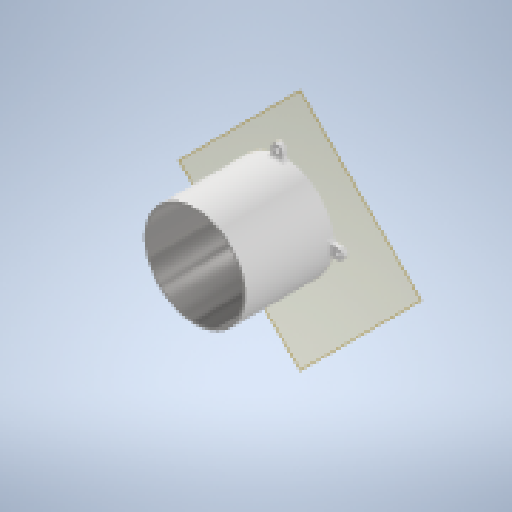
# Autodesk Inventor part: Camisa
Saved by Autodesk Inventor 2023 (Build 270158000, 158)
## iProperties
Created: 2022-11-24
Part Number: Camisa
Material: Genérico
Document SubType Name: Modeling
Designer: sergi
Density: 1 g/cm^3
Appearance: Valor por defecto
Author: sergi
Autodesk Inventor part; units mm, degrees
ref_plane "YZ Plane" through (0, 0, 0) normal (1, 0, 0) x (0, 1, 0)
ref_plane "XZ Plane" through (0, 0, 0) normal (0, 1, 0) x (-1, 0, 0)
ref_plane "XY Plane" through (0, 0, 0) normal (0, 0, 1) x (1, 0, 0)
ref_plane "Plano de trabajo1" through (0, 0, 0) normal (0, 0, 1) x (1, 0, 0)
sketch "Boceto1" plane through (0, 0, 0) normal (0, 0, 1) x (1, 0, 0)
  arc A0 (29.505692, -74.908522) -> (70.494308, -74.908522) centre (50, -53) ccw
  circle A1 centre (50, -53) radius 30
  circle A2 centre (50, -53) radius 31.5
  point P0 (0, 0)
  dimension "d0" = 60
  dimension "d1" = 63
  constraints: 2 centre point, 2 coincident
  measures "d0" diameter of A1
  measures "d1" diameter of A2
extrude "Extrusión1" add sketch "Boceto1" along normal blind 55
ref_plane "Plano de trabajo2" through (38.332738, -41.332738, 0) normal (0, 0, 1) x (0.7071068, 0.7071068, 0)
sketch "Boceto3" plane through (38.332738, -41.332738, 0) normal (0, 0, 1) x (0.7071068, 0.7071068, 0)
  circle A0 centre (25.37, -43.5) radius 1.25
  arc A1 (23.001522, -45.725492) -> (27.738478, -41.274508) centre (25.37, -43.5) ccw
  line L0 (-2.057062, -23.435368) -> (-6.794017, -18.984385)
  circle A2 centre (-25.37, -43.5) radius 1.25
  arc A3 (-27.738478, -41.274508) -> (-23.001522, -45.725492) centre (-25.37, -43.5) ccw
  line L1 (0, -16.5) -> (-25.37, -43.5)
  arc A4 (-17.377185, -42.773246) -> (-20.578232, -43.146507) centre (-18.756326, -44.858424) ccw
  arc A5 (-25.315188, -38.695524) -> (-25.141719, -35.47746) centre (-27.137093, -36.983607) ccw
  line L2 (25.37, -43.5) -> (0, -16.5)
  arc A6 (20.578232, -43.146507) -> (17.377185, -42.773246) centre (18.756326, -44.858424) ccw
  arc A7 (25.141719, -35.47746) -> (25.315188, -38.695524) centre (27.137093, -36.983607) ccw
  line L3 (23.001522, -45.725492) -> (20.578232, -43.146507)
  line L4 (19.086559, -41.558996) -> (3.55069, -25.024961)
  line L5 (27.738478, -41.274508) -> (25.315188, -38.695524)
  line L6 (23.823514, -37.108012) -> (8.109422, -20.384303)
  line L7 (-3.008681, -24.448128) -> (-19.086559, -41.558996)
  line L8 (-20.578232, -43.146507) -> (-23.001522, -45.725492)
  line L9 (-6.794017, -18.984385) -> (-23.823514, -37.108012)
  line L10 (-25.315188, -38.695524) -> (-27.738478, -41.274508)
  line L11 (0, -16.5) -> (23.823514, -16.5)
  arc A8 (-21.522288, 12.642227) -> (-27.747366, 6.792958) centre (-24.634827, 9.717593) ccw
  line L12 (1.388517, -10.426349) -> (6.125473, -14.877333)
  arc A9 (27.069933, 7.412791) -> (22.183049, 12.004652) centre (24.626491, 9.708721) ccw
  line L13 (0, -16.5) -> (24.626491, 9.708721)
  line L14 (-24.634827, 9.717593) -> (0, -16.5)
  line L15 (-21.522288, 12.642227) -> (-17.698076, 8.572314)
  line L16 (-17.607324, 8.475731) -> (-2.071456, -8.058304)
  line L17 (-27.747366, 6.792958) -> (-25.324076, 4.213974)
  line L18 (-23.832403, 2.626462) -> (-8.118311, -14.097247)
  line L19 (-1.356721, -13.047528) -> (14.721157, 4.06334)
  line L20 (14.901827, 4.255618) -> (22.183049, 12.004652)
  line L21 (6.125473, -14.877333) -> (23.15497, 3.246294)
  line L22 (24.646643, 4.833806) -> (27.069933, 7.412791)
  circle A10 centre (-24.626491, 9.708721) radius 1.25
  circle A11 centre (0, -16.5) radius 31.5
  circle A12 centre (24.626491, 9.708721) radius 1.25
  circle A13 centre (-27.750165, 3.145059) radius 2.5
  circle A14 centre (-17.881275, 12.418161) radius 2.5
  circle A15 centre (27.19986, 3.900187) radius 2.5
  circle A16 centre (18.669164, 11.915881) radius 2.5
  circle A17 centre (0, -16.5) radius 31.5
  point P0 (2.12132, 56.331998)
  point P1 (17.377185, -42.773246)
  point P2 (-25.141719, -35.47746)
  point P3 (-17.377185, -42.773246)
  point P4 (-16.566475, 10.291825)
  point P5 (-19.70318, 10.706244)
  point P6 (-25.928259, 4.856975)
  point P7 (-25.709712, 1.700569)
  point P8 (25.19987, 2.400173)
  point P9 (25.377954, 5.612103)
  point P10 (20.49107, 10.203965)
  point P11 (17.296431, 9.826478)
  dimension "d18" = 2
  dimension "d24" = 6.5
  dimension "d26" = 2
  dimension "d28" = 5
  dimension "d29" = 5
  dimension "d30" = 5
  dimension "d31" = 5
  dimension "d35" = 6.5
  dimension "d40" = 2.5
  dimension "d41" = 2.5
  dimension "d42" = 5
  dimension "d43" = 5
  dimension "d44" = 5
  dimension "d45" = 5
  constraints: 46 end point, 28 tangent, 20 parallel, 16 point on circle, 14 centre point, 2 coincident, 1 horizontal, 1 point on line, 8 other
  measures "d18" radial gap between concentric circles of A0 A1
  measures "d24" distance of L0.start L0.end
  measures "d26" radial gap between concentric circles of A2 A3
  measures "d28" diameter of A4
  measures "d29" diameter of A5
  measures "d30" diameter of A6
  measures "d31" diameter of A7
  measures "d35" distance of L12.start L12.end
  measures "d40" diameter of A10
  measures "d41" diameter of A12
  measures "d42" diameter of A13
  measures "d43" diameter of A14
  measures "d44" diameter of A15
  measures "d45" diameter of A16
extrude "Extrusión3" add sketch "Boceto3" along normal blind 3 contours L3 A6 A11 A7 L5 A1 | A4 L8 A3 L10 A5 A11 | A11 L20 A9 L22 A15 | A11 A13 L17 A8 L15 | A11 A16 L20 | L15 A14 A11
fillet "Empalme2" radius 2 5 edges at (50.98, -84.4848, 3) (81.4242, -50.8153, 3) (81.341, -56.1612, 3) (49.02, -21.5152, 3) (18.5152, -52.02, 3)
